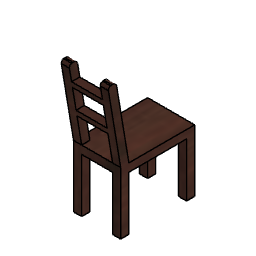
Exp 6.2 (Autodesk Fusion 360 design; units mm, degrees)
Autodesk Fusion 360 part; units mm, degrees
sketch "Sketch1" plane through (0, 0, 0) normal (0, 1, 0) x (1, 0, 0)
  line L0 (0, 0) -> (-35, 0)
  line L1 (-35, 0) -> (-35, -6)
  line L2 (-35, -6) -> (0, -6)
  line L3 (0, -6) -> (0, 0)
  dimension "d1" = 35
  dimension "d2" = 6
  constraint horizontal L0
  constraint vertical L1
  constraint horizontal L2
  constraint vertical L3
  constraint coincident L0.start L3.end
  measures "d1" distance of L0.start L0.end
  measures "d2" distance of L0.start L2.end
extrude "Extrude1" add sketch "Sketch1" along normal blind 55
sketch "Sketch2" plane through (0, 0, 0) normal (0, 0, -1) x (1, 0, 0)
  line L0 (0, 0) -> (-35, 0)
  line L1 (-35, 0) -> (-35, -55)
  line L2 (-35, -55) -> (0, -55)
  line L3 (0, -55) -> (0, 0)
  line L4 (-35, 0) -> (-29, 0)
  line L5 (-29, 0) -> (-29, -6)
  line L6 (-29, -6) -> (-35, -6)
  line L7 (-35, 0) -> (-35, -6)
  line L8 (0, 0) -> (0, -6)
  line L9 (0, -6) -> (-6, -6)
  line L10 (-6, 0) -> (-6, -6)
  line L11 (-6, 0) -> (0, 0)
  line L12 (-35, -24.5) -> (-35, -30.5)
  line L13 (0, -24.5) -> (0, -30.5)
  line L14 (-29, -49) -> (-29, -55)
  line L15 (-29, -55) -> (-35, -55)
  line L16 (-35, -49) -> (-35, -55)
  line L17 (-35, -49) -> (-29, -49)
  line L18 (0, -49) -> (0, -55)
  line L19 (0, -55) -> (-6, -55)
  line L20 (-6, -49) -> (-6, -55)
  line L21 (-6, -49) -> (0, -49)
  dimension "d8" = 29
  dimension "d9" = -49
  constraint coincident L0.end L1.start
  constraint coincident L0 L4.end
  constraint perpendicular L1 L4
  constraint perpendicular L4 L5
  constraint coincident L1 L6.end
  constraint perpendicular L1 L6
extrude "Extrude2" add sketch "Sketch2" along normal blind 40 contours L0 L3 L8 L9 L10 L11 | L0 L1 L4 L5 L6 L7 | L2 L3 L18 L19 L20 L21 | L1 L2 L14 L15 L16 L17
sketch "Sketch3" plane through (0, 0, 0) normal (1, 0, 0) x (0, 1, 0)
  line L0 (0, 6) -> (0, -40)
  line L1 (0, -40) -> (6, -40)
  line L2 (6, -40) -> (6, 0)
  line L3 (6, 0) -> (49, 0)
  line L4 (49, 0) -> (49, -40)
  line L5 (49, -40) -> (55, -40)
  line L6 (55, -40) -> (55, 6)
  line L7 (55, 6) -> (0, 6)
  line L8 (0, 6) -> (-9.4363, 62)
  line L9 (-9.4363, 62) -> (-3.5197, 62.997)
  line L10 (-3.5197, 62.997) -> (6.0846, 6)
  line L11 (0, 6) -> (6.0846, 6)
  dimension "d14" = 6
  constraint coincident L0.start L7.end
  constraint perpendicular L8 L9
  constraint coincident L7 L10.end
  constraint parallel L8 L10
  measures "d14" distance of L8.end L9.end
extrude "Extrude3" add sketch "Sketch3" against normal blind 6 contours L7 L8 L9 L10 L11
fillet "Fillet1" radius 3 1 edges at (-3, -3.5197, 62.997)
fillet "Fillet2" radius 2 1 edges at (-3, -9.4363, 62)
pattern_linear "R-Pattern1" count 1 spacing 0 along (0, 0, -1) count 2 spacing 29 along (-1, 0, 0) of "Extrude3", "Fillet1", "Fillet2"
sketch "Sketch5" plane through (-29, 0, 0) normal (1, 0, 0) x (0, 1, 0)
  arc A0 (-7.4641, 62.3323) -> (-9.104, 60.0278) centre (-7.1318, 60.3601) ccw
  line L0 (-9.104, 60.0278) -> (0, 6)
  line L1 (0, 6) -> (6.0846, 6)
  line L2 (6.0846, 6) -> (-3.0213, 60.0387)
  arc A1 (-3.0213, 60.0387) -> (-6.478, 62.4985) centre (-5.9795, 59.5402) ccw
  line L3 (-6.478, 62.4985) -> (-7.4641, 62.3323)
  line L4 (-7.4983, 50.4985) -> (-1.4137, 50.4985)
  line L5 (-7.4983, 50.4985) -> (-6.8242, 46.4985)
  line L6 (-6.8242, 46.4985) -> (-0.7396, 46.4985)
  line L7 (-1.4137, 50.4985) -> (-0.7396, 46.4985)
  line L8 (-4.1281, 30.4985) -> (1.9564, 30.4985)
  line L9 (-3.4541, 26.4985) -> (2.6305, 26.4985)
  line L10 (-4.1281, 30.4985) -> (-3.4541, 26.4985)
  line L11 (1.9564, 30.4985) -> (2.6305, 26.4985)
  constraint coincident L0 L4.start
  constraint coincident L2 L4.end
  constraint horizontal L4
  constraint coincident L0 L5.end
  constraint parallel L0 L5
  constraint coincident L2 L6.end
  constraint parallel L4 L6
  constraint parallel L2 L7
  constraint coincident L0 L8.start
  constraint coincident L2 L8.end
  constraint horizontal L8
  constraint coincident L0 L9.start
  constraint coincident L2 L9.end
  constraint parallel L8 L9
  constraint parallel L0 L10
  constraint parallel L2 L11
extrude "Extrude4" add sketch "Sketch5" along normal blind 23 contours L0 L2 L4 L5 L6 L7 | L0 L2 L8 L9 L10 L11
equation "d3 = 43 mm + 6 mm + 6 mm"
